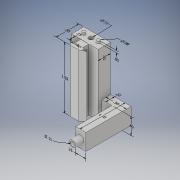
# Autodesk Inventor part: Grab1
Saved by Autodesk Inventor 2018 (Build 220112000, 112)
## iProperties
Created: 2019-12-05
Part Number: Grab1
Material: Generic
Document SubType Name: Modeling
Designer: AOFUser
Density: 1 g/cm^3
Appearance: Default
Author: AOFUser
Autodesk Inventor part; units mm, degrees
ref_plane "YZ Plane" through (0, 0, 0) normal (1, 0, 0) x (0, 1, 0)
ref_plane "XZ Plane" through (0, 0, 0) normal (0, 1, 0) x (-1, 0, 0)
ref_plane "XY Plane" through (0, 0, 0) normal (0, 0, 1) x (1, 0, 0)
sketch "Sketch1" plane through (0, 0, 0) normal (0, 1, 0) x (-1, 0, 0)
  line L0 (0, 0) -> (-16.51, 0)
  line L1 (-16.51, 0) -> (-16.51, -7.62)
  line L2 (-16.51, -7.62) -> (0, -7.62)
  line L3 (0, -7.62) -> (0, 0)
  line L4 (-8.255, 0) -> (-5.715, 0)
  line L5 (-5.715, 0) -> (-5.715, 6.35)
  line L6 (-5.715, 6.35) -> (-10.795, 6.35)
  line L7 (-10.795, 6.35) -> (-10.795, 0)
  line L8 (-5.715, -7.62) -> (-5.715, -8.89)
  line L9 (-5.715, -8.89) -> (-10.795, -8.89)
  line L10 (-10.795, -8.89) -> (-10.795, -7.62)
  line L11 (-10.795, 6.35) -> (-10.795, 3.81)
  line L12 (-10.795, 3.81) -> (-13.335, 3.81)
  line L13 (-13.335, 3.81) -> (-10.795, 6.35)
  line L14 (-5.715, 6.35) -> (-5.715, 3.81)
  line L15 (-5.715, 3.81) -> (-3.175, 3.81)
  line L16 (-3.175, 3.81) -> (-5.715, 6.35)
  point P0 (-8.255, -7.62)
  point P1 (0, -3.81)
  point P2 (-16.51, -3.81)
  dimension "d0" = 16.51
  dimension "d1" = 7.62
  dimension "d2" = 2.54
  dimension "d3" = 6.35
  dimension "d4" = 5.08
  dimension "d5" = 1.27
  dimension "d6" = 2.54
  dimension "d7" = 2.54
  dimension "d8" = 2.54
  dimension "d9" = 2.54
  constraints: 34 end point, 10 point on line, 5 perpendicular, 4 midpoint, 3 parallel, 2 coincident, 2 horizontal
  measures "d0" distance of L2.end L1.end
  measures "d1" distance of L1.end L0.end
  measures "d2" distance of L4.start L4.end
  measures "d3" distance of L4.end L5.end
  measures "d4" distance of L5.end L6.end
  measures "d5" distance of L8.start L8.end
  measures "d6" distance of L6.end L11.end
  measures "d7" distance of L11.end L12.end
  measures "d8" distance of L5.end L14.end
  measures "d9" distance of L14.end L15.end
extrude "Extrusion1" add sketch "Sketch1" along normal blind 38.1
sketch "Sketch2" plane through (0, 38.1, 0) normal (0, 1, 0) x (1, 0, 0)
  line L0 (16.51, 0) -> (16.51, 7.62) projected
  line L1 (16.51, 3.81) -> (12.7, 3.81)
  line L2 (0, 7.62) -> (0, 0) projected
  circle A0 centre (12.7, 3.81) radius 1.016
  dimension "d12" = 3.81
  dimension "d14" = 2.032
  constraints: 2 end point, 1 centre point, 1 coincident, 1 horizontal, 1 midpoint
  measures "d12" distance of L1.start L1.end
  measures "d14" diameter of A0
extrude "Extrusion2" add sketch "Sketch2" along normal blind 1.27
sketch "Sketch3" plane through (0, 38.1, 0) normal (0, 1, 0) x (1, 0, 0)
  line L0 (0, 7.62) -> (0, 0) projected
  line L1 (0, 3.81) -> (3.81, 3.81)
  circle A0 centre (3.81, 3.81) radius 1.016
  dimension "d20" = 3.81
  dimension "d21" = 2.032
  constraints: 2 end point, 1 centre point, 1 coincident, 1 horizontal, 1 midpoint
  measures "d20" distance of L1.start L1.end
  measures "d21" diameter of A0
extrude "Extrusion3" add sketch "Sketch3" along normal blind 1.27
sketch "Sketch6" plane through (0, 38.1, 0) normal (0, 1, 0) x (1, 0, 0)
  line L0 (16.51, 0) -> (16.51, 7.62) projected
  line L1 (16.51, 3.81) -> (8.255, 3.81)
  circle A0 centre (8.255, 3.81) radius 1.397
  point P0 (0, 0)
  dimension "d24" = 8.255
  dimension "d25" = 2.794
  constraints: 2 end point, 1 centre point, 1 coincident, 1 horizontal, 1 midpoint
  measures "d24" distance of L1.start L1.end
  measures "d25" diameter of A0
hole "Hole1" at (8.255, 38.1, -3.81) at (8.255, 38.1, -3.81) direction (0, -1, 0) diameter 2.794 depth 11.43 tip angle 118
sketch "Sketch7" plane through (16.51, 0, 0) normal (1, 0, 0) x (0, 0, -1)
  line L0 (0, 0) -> (7.62, 0) projected
  line L1 (7.62, 0) -> (2.159, 0)
  line L2 (2.159, 0) -> (2.159, 10.16)
  line L3 (2.159, 10.16) -> (7.62, 10.16)
  line L4 (7.62, 10.16) -> (7.62, 0)
  dimension "d33" = 5.461
  dimension "d34" = 10.16
  constraints: 8 end point, 2 parallel, 1 horizontal, 1 perpendicular
  measures "d33" distance of L2.end L3.end
  measures "d34" distance of L1.end L2.end
extrude "Extrusion4" add sketch "Sketch7" along normal blind 12.7
sketch "Sketch8" plane through (16.51, 0, -2.159) normal (0, 0, 1) x (1, 0, 0)
  line L0 (12.7, 0) -> (12.7, 10.16) projected
  line L1 (0, 10.16) -> (12.7, 10.16) projected
  line L2 (12.7, 0) -> (6.35, 0)
  line L3 (6.35, 0) -> (6.35, 10.16)
  line L4 (6.35, 10.16) -> (12.7, 10.16)
  line L5 (12.7, 10.16) -> (12.7, 0)
  point P0 (-16.51, 0)
  constraints: 8 end point, 2 parallel, 1 horizontal, 1 midpoint, 1 perpendicular
extrude "Extrusion5" add sketch "Sketch8" along normal blind 22.479
sketch "Sketch11" plane through (16.51, 0, 20.32) normal (0, 0, 1) x (1, 0, 0)
  line L0 (12.7, 0) -> (12.7, 10.16) projected
  line L1 (12.7, 5.08) -> (9.525, 5.08)
  circle A0 centre (9.525, 5.08) radius 2.032
  point P0 (-16.51, 0)
  dimension "d41" = 3.175
  dimension "d42" = 4.064
  constraints: 2 end point, 1 centre point, 1 coincident, 1 horizontal, 1 midpoint
  measures "d41" distance of L1.start L1.end
  measures "d42" diameter of A0
extrude "Extrusion6" add sketch "Sketch11" along normal blind 5.08
sketch "Sketch12" plane through (26.035, 5.08, 25.4) normal (0, 0, 1) x (1, 0, 0)
  circle A0 centre (0, 0) radius 1.397
  point P0 (-26.035, -5.08)
  dimension "d45" = 2.794
  constraints: 1 centre point
  measures "d45" diameter of A0
hole "Hole2" at (26.035, 5.08, 25.4) direction (0, 0, -1) diameter 2.794 depth 12.7 tip angle 118
sketch "Sketch13" plane through (10.795, 0, -8.89) normal (0, 0, -1) x (-1, 0, 0)
  line L0 (0, 0) -> (0, 38.1) projected
  line L1 (0, 0) -> (5.08, 0) projected
  line L2 (0, 38.1) -> (5.08, 38.1)
  line L3 (5.08, 38.1) -> (5.08, 0)
  line L4 (5.08, 0) -> (0, 0)
  line L5 (0, 0) -> (0, 38.1)
  point P0 (10.795, 0)
  constraints: 8 end point, 2 parallel, 1 horizontal, 1 perpendicular
extrude "Extrusion7" cut sketch "Sketch13" against normal blind 1.27
body "Solid1"
